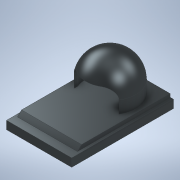
# Autodesk Inventor part: каска
Saved by Autodesk Inventor 2020.1 (Build 241239000, 239)
## iProperties
Created: 2022-03-19
Part Number: каска
Material: Чугун, серый
Document SubType Name: Modeling
Designer: User
Density: 7.15 g/cm^3
Appearance: Чугун серый
Author: User
Autodesk Inventor part; units mm, degrees
ref_plane "YZ Plane" through (0, 0, 0) normal (1, 0, 0) x (0, 1, 0)
ref_plane "XZ Plane" through (0, 0, 0) normal (0, 1, 0) x (-1, 0, 0)
ref_plane "XY Plane" through (0, 0, 0) normal (0, 0, 1) x (1, 0, 0)
sketch "Эскиз1" plane through (0, 0, 0) normal (0, 1, 0) x (-1, 0, 0)
  circle A0 centre (0, 0) radius 60
  circle A1 centre (0, 0) radius 64
  line L0 (64, 0) -> (-64, 0)
  point P0 (60, 0)
  point P1 (-60, 0)
  dimension "d0" = 120
  dimension "d1" = 128
  constraints: 2 centre point, 2 coincident, 2 end point, 2 point on circle, 1 horizontal
  measures "d0" diameter of A0
  measures "d1" diameter of A1
revolve "Вращение1" add sketch "Эскиз1" angle 180 about axis through (-64, 0, 0) along (1, 0, 0) picked at (62.0387, -7.1775) contours L0 A1 A0
sketch "Эскиз2" plane through (0, 0, 0) normal (0, 0, 1) x (1, 0, 0)
  line L0 (-64, 0) -> (64, 0) projected
  circle A0 centre (-30, 0) radius 25
  circle A1 centre (30, 0) radius 25
  line L1 (-30, 25) -> (30, 25)
  point P0 (0, 0)
  point P1 (0, 0)
  point P2 (55, 0)
  point P3 (-55, 0)
  dimension "d3" = 50
  dimension "d4" = 50
  dimension "d5" = 30
  dimension "d6" = 30
  constraints: 2 end point, 2 point on line, 1 coincident, 1 horizontal, 6 other
  measures "d5" distance of point (0, 0) point (-30, 0)
  measures "d6" distance of point (0, 0) point (30, 0)
extrude "Выдавливание1" cut sketch "Эскиз2" along normal blind 100 contours A0 L0 | A0 L1 A1 L0 | A1 L0 picked at (-26.3843, 7.5081) picked at (33.6157, 7.5081)
sketch "Эскиз3" plane through (0, 0, 0) normal (0, -1, 0) x (1, 0, 0)
  circle A0 centre (0, 0) radius 64
  circle A1 centre (0, 0) radius 60
  arc A2 (-55, 23.9792) -> (55, 23.9792) centre (0, 0) ccw projected
  arc A3 (-55, 32.7261) -> (55, 32.7261) centre (0, 0) ccw projected
  line L0 (55, 23.9792) -> (55, 32.7261)
  line L1 (-55, 23.9792) -> (-55, 32.7261) projected
  line L2 (-55, 23.9792) -> (-55, 32.7261)
  constraints: 4 end point, 2 centre point, 2 coincident, 2 vertical, 1 point on circle
extrude "Выдавливание2" add sketch "Эскиз3" along normal blind 30 contours A0 L1 A1 L0 picked at (62.3402, -3.7177)
sketch "Эскиз5" plane through (0, -30, 0) normal (0, -1, 0) x (1, 0, 0)
  line L0 (-73.6951, -73.9104) -> (73.6951, -73.9104)
  line L1 (73.6951, -73.9104) -> (73.6951, 153.3574)
  line L2 (73.6951, 153.3574) -> (-73.6951, 153.3574)
  line L3 (-73.6951, 153.3574) -> (-73.6951, -73.9104)
  line L4 (0, 153.3574) -> (0, -73.9104)
  point P0 (0, 0)
  constraints: 10 end point, 2 midpoint, 2 parallel, 2 perpendicular, 1 horizontal, 1 other
extrude "Выдавливание3" add sketch "Эскиз5" along normal blind 10
chamfer "Фаска1" distance 10 angle 45 1 edges at (0, -30, 153.3574)
sketch "Эскиз6" plane through (0, -40, 0) normal (0, -1, 0) x (1, 0, 0)
  line L0 (-80, -76.0724) -> (80, -76.0724)
  line L1 (80, -76.0724) -> (80, 173.9276)
  line L2 (80, 173.9276) -> (-80, 173.9276)
  line L3 (-80, 173.9276) -> (-80, -76.0724)
  line L4 (0, 173.9276) -> (0, -76.0724)
  point P0 (0, 0)
  dimension "d16" = 160
  dimension "d17" = 250
  constraints: 10 end point, 2 midpoint, 2 parallel, 2 perpendicular, 1 horizontal, 1 other
  measures "d16" distance of L0.start L0.end
  measures "d17" distance of L0.end L1.end
extrude "Выдавливание4" add sketch "Эскиз6" along normal blind 20
